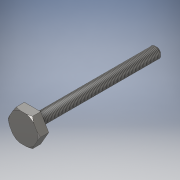
# Autodesk Inventor part: HexBoltAJB
Saved by Autodesk Inventor 2018 (Build 220112000, 112)
## iProperties
Created: 2018-02-03
Part Number: HexBoltAJB
Material: Iron, Malleable
Document SubType Name: Modeling
Designer: Alec temporary
Density: 7.15 g/cm^3
Appearance: Semi-Polished
Author: Alec temporary
Autodesk Inventor part; units mm, degrees
ref_plane "YZ Plane" through (0, 0, 0) normal (1, 0, 0) x (0, 1, 0)
ref_plane "XZ Plane" through (0, 0, 0) normal (0, 1, 0) x (-1, 0, 0)
ref_plane "XY Plane" through (0, 0, 0) normal (0, 0, 1) x (1, 0, 0)
sketch "Sketch1" plane through (0, 0, 0) normal (0, 0, 1) x (1, 0, 0)
  circle A0 centre (0, 0) radius 11.1125
  dimension "d0" = 22.225
  constraints: 1 centre point, 1 coincident
  measures "d0" diameter of A0
extrude "Extrusion1" add sketch "Sketch1" along normal blind 255.27
sketch "Sketch2" plane through (0, 0, 255.27) normal (0, 0, 1) x (1, 0, 0)
  line L0 (16.6687, 28.8711) -> (33.3375, 0)
  line L1 (33.3375, 0) -> (16.6687, -28.8711)
  line L2 (16.6687, -28.8711) -> (-16.6688, -28.8711)
  line L3 (-16.6688, -28.8711) -> (-33.3375, 0)
  line L4 (-33.3375, 0) -> (-16.6688, 28.8711)
  line L5 (-16.6688, 28.8711) -> (16.6687, 28.8711)
  circle A0 centre (0, 0) radius 11.1125 construction
  dimension "d3" = 33.3375
  dimension "d6" = 22.225
  constraints: 12 end point, 1 coincident, 1 horizontal, 13 other
  measures "d3" distance of L1.end L2.end
  measures "d6" diameter of A0
extrude "Extrusion2" add sketch "Sketch2" along normal blind 19.05
sketch "Sketch3" plane through (0, 0, 0) normal (0, 1, 0) x (-1, 0, 0)
  line L0 (33.3375, 274.32) -> (16.6687, 274.32) projected
  line L1 (29.5275, 274.32) -> (33.3375, 271.78)
  line L2 (33.3375, 271.78) -> (33.3375, 274.32)
  line L3 (33.3375, 274.32) -> (29.5275, 274.32)
  line L4 (0, -55.626) -> (0, 333.756) projected
  point P0 (0, 0)
  dimension "d7" = 2.54
  dimension "d8" = 3.81
  constraints: 6 end point, 1 collinear, 1 perpendicular, 1 point on line
  measures "d7" distance of L1.end L0.start
  measures "d8" distance of L0.start L1.start
revolve "Revolution1" cut sketch "Sketch3" angle 360 about axis through (0, 0, -10) along (0, 0, 1)
sketch "Sketch4" plane through (0, 0, 255.27) normal (0, 0, -1) x (-1, 0, 0)
  circle A0 centre (0, 0) radius 22.225
  dimension "d10" = 44.45
  constraints: 1 centre point, 1 coincident
  measures "d10" diameter of A0
extrude "Extrusion3" add sketch "Sketch4" along normal blind 1.27
chamfer "Chamfer1" distance 3.175 angle 45 1 edges at (-11.1125, 0, 0)
thread "Thread1" size "7/8-9 UNC" class "2A" standard "ANSI Unified Screw Threads" full length
equation "\"d3\" = 1.5 * d6"
body "Solid1"
